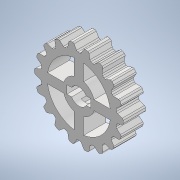
# Autodesk Inventor part: center_gear
Saved by Autodesk Inventor 2022 (Build 260153000, 153)
## iProperties
Created: 2022-06-21
Part Number: center_gear
Material: Generic
Document SubType Name: Modeling
Designer: efred
Density: 1 g/cm^3
Appearance: Default
Author: efred
Autodesk Inventor part; units mm, degrees
ref_plane "YZ Plane" through (0, 0, 0) normal (1, 0, 0) x (0, 1, 0)
ref_plane "XZ Plane" through (0, 0, 0) normal (0, 1, 0) x (-1, 0, 0)
sketch "Sketch1" plane through (0, 0, 0) normal (0, 0, 1) x (1, 0, 0)
  circle A0 centre (0, 0) radius 0.5 projected
  line L0 (-1.1547, -2) -> (-1.7321, -1) projected
  line L1 (-1.7321, -1) -> (-3.5, -1) projected
  line L2 (-3.5, -1) -> (-3.5, 1) projected
  line L3 (-3.5, 1) -> (-1.7321, 1) projected
  line L4 (-1.7321, 1) -> (-1.1547, 2) projected
  line L5 (-1.1547, 2) -> (1.1547, 2) projected
  line L6 (1.1547, 2) -> (1.7321, 1) projected
  line L7 (1.7321, 1) -> (3.5, 1) projected
  line L8 (3.5, 1) -> (3.5, -1) projected
  line L9 (3.5, -1) -> (1.7321, -1) projected
  line L10 (1.7321, -1) -> (1.1547, -2) projected
  line L11 (1.1547, -2) -> (-1.1547, -2) projected
  circle A1 centre (0, 0) radius 5
  line L12 (-3.8, -1.3) -> (-1.9053, -1.3)
  line L13 (-1.9053, -1.3) -> (-1.3279, -2.3)
  line L14 (-1.3279, -2.3) -> (1.3279, -2.3)
  line L15 (1.3279, -2.3) -> (1.9053, -1.3)
  line L16 (1.9053, -1.3) -> (3.8, -1.3)
  line L17 (3.8, -1.3) -> (3.8, 1.3)
  line L18 (3.8, 1.3) -> (1.9053, 1.3)
  line L19 (1.9053, 1.3) -> (1.3279, 2.3)
  line L20 (1.3279, 2.3) -> (-1.3279, 2.3)
  line L21 (-1.3279, 2.3) -> (-1.9053, 1.3)
  line L22 (-1.9053, 1.3) -> (-3.8, 1.3)
  line L23 (-3.8, 1.3) -> (-3.8, -1.3)
  dimension "d0" = 10
  dimension "d1" = 0.3
  constraints: 24 end point, 1 centre point, 1 coincident, 11 other
  measures "d0" diameter of A1
  measures "d1" distance between parallel lines of L1 L12
extrude "Extrusion1" add sketch "Sketch1" along normal blind 2 and the other way blind 5 contours A1
sketch "Sketch2" plane through (0, 0, -5) normal (0, 0, -1) x (-1, 0, 0)
  circle A0 centre (0, 0) radius 5 projected
  line L0 (3.8, 1.3) -> (3.8, -1.3) projected
  line L1 (3.8, -1.3) -> (1.9053, -1.3) projected
  line L2 (1.9053, -1.3) -> (1.3279, -2.3) projected
  line L3 (1.3279, -2.3) -> (-1.3279, -2.3) projected
  line L4 (-1.3279, -2.3) -> (-1.9053, -1.3) projected
  line L5 (-1.9053, -1.3) -> (-3.8, -1.3) projected
  line L6 (-3.8, -1.3) -> (-3.8, 1.3) projected
  line L7 (-3.8, 1.3) -> (-1.9053, 1.3) projected
  line L8 (-1.9053, 1.3) -> (-1.3279, 2.3) projected
  line L9 (-1.3279, 2.3) -> (1.3279, 2.3) projected
  line L10 (1.3279, 2.3) -> (1.9053, 1.3) projected
  line L11 (1.9053, 1.3) -> (3.8, 1.3) projected
  line L12 (3.8, 1.3) -> (3.8, -1.3) projected
  line L13 (3.8, 1.3) -> (3.8, -1.3)
  line L14 (3.8, -1.3) -> (1.9053, -1.3)
  line L15 (1.9053, -1.3) -> (1.3279, -2.3) projected
  line L16 (1.9053, -1.3) -> (1.3279, -2.3)
  line L17 (-1.9053, -1.3) -> (-1.3279, -2.3) projected
  line L18 (-1.3279, -2.3) -> (1.3279, -2.3)
  line L19 (1.9053, 1.3) -> (3.8, 1.3) projected
  line L20 (3.8, 1.3) -> (1.9053, 1.3)
  line L21 (1.3279, 2.3) -> (1.9053, 1.3) projected
  line L22 (1.9053, 1.3) -> (1.3279, 2.3)
  line L23 (1.3279, 2.3) -> (-1.3279, 2.3)
  line L24 (-1.3, 1.9053) -> (-2.3, 1.3279)
  line L25 (-2.3, 1.3279) -> (-2.3, -1.3279)
  line L26 (2.3, -1.3279) -> (2.3, 1.3279)
  line L27 (1.3, 1.9053) -> (2.3, 1.3279)
  line L28 (1.3, 3.8) -> (1.3, 1.9053)
  line L29 (-1.3, 3.8) -> (-1.3, 1.9053)
  line L30 (-1.3, 3.8) -> (1.3, 3.8)
  line L31 (-1.9053, -1.3) -> (-1.3279, -2.3)
  line L32 (-1.3279, -2.3) -> (1.3279, -2.3)
  line L33 (1.3279, 2.3) -> (-1.3279, 2.3)
  line L34 (-1.9053, 1.3) -> (-1.3279, 2.3)
  line L35 (-3.8, 1.3) -> (-1.9053, 1.3)
  line L36 (-3.8, -1.3) -> (-1.9053, -1.3)
  line L37 (-3.8, -1.3) -> (-3.8, 1.3)
  line L38 (1.3, -1.9053) -> (2.3, -1.3279)
  line L39 (2.3, -1.3279) -> (2.3, 1.3279)
  line L40 (-2.3, 1.3279) -> (-2.3, -1.3279)
  line L41 (-1.3, -1.9053) -> (-2.3, -1.3279)
  line L42 (-1.3, -3.8) -> (-1.3, -1.9053)
  line L43 (1.3, -3.8) -> (1.3, -1.9053)
  line L44 (1.3, -3.8) -> (-1.3, -3.8)
  point P0 (1.3, -2.3)
  point P1 (-1.3, -2.3)
  point P2 (-1.3, 2.3)
  point P3 (1.3, 2.3)
  point P4 (-2.3, 1.3)
  point P5 (-1.6837, 1.6837)
  point P6 (-1.6837, -1.6837)
  point P7 (-2.3, -1.3)
  point P8 (1.6837, -1.6837)
  point P9 (2.3, -1.3)
  point P10 (1.6837, 1.6837)
  point P11 (2.3, 1.3)
  dimension "d8" = 360
  constraints: 56 end point, 4 collinear, 1 point on line, 65 other
ref_plane "Work Plane1" through (-8.8, -2.2, 0) normal (0, 0, 1) x (1, 0, 0)
extrude "Extrusion2" cut sketch "Sketch2" against normal up to surface (5 mm away) contours L11 L10 L27 L26 | L26 L38 L2 L1 | L9 L29 L30 L28 | L43 L44 L42 L3 | L8 L7 L25 L24 | L41 L25 L5 L4
sketch "Sketch3" plane through (0, 0, -5) normal (0, 0, -1) x (-1, 0, 0)
  line L0 (-1.6837, 1.6837) -> (-2.3, 1.3279) projected
  circle A0 centre (0, 0) radius 2.6558
  constraints: 1 coincident, 3 other
extrude "Extrusion3" cut sketch "Sketch3" against normal through all
sketch "Sketch4" plane through (0, 0, -5) normal (0, 0, -1) x (-1, 0, 0)
  circle A0 centre (0, 0) radius 5 projected
  circle A1 centre (0, 0) radius 14.5 construction
  circle A2 centre (-20.3143, -27.9603) radius 16.5 construction
  circle A3 centre (0, 0) radius 12.5
  circle A4 centre (0, 0) radius 10.5
  line L0 (-12.4097, -1.5) -> (-4.7697, -1.5)
  line L1 (-4.7697, -1.5) -> (-4.7697, 1.5)
  line L2 (-4.7697, 1.5) -> (-12.4097, 1.5)
  line L3 (-12.4097, 1.5) -> (-12.4097, -1.5)
  line L4 (-5, 0) -> (-10.5, 0) construction
  line L5 (1.5, -12.4097) -> (1.5, -4.7697)
  line L6 (-1.5, -4.7697) -> (-1.5, -12.4097)
  line L7 (12.4097, 1.5) -> (4.7697, 1.5)
  line L8 (4.7697, -1.5) -> (12.4097, -1.5)
  line L9 (-1.5, 12.4097) -> (-1.5, 4.7697)
  line L10 (1.5, 4.7697) -> (1.5, 12.4097)
  line L11 (-14.1647, -0.8644) -> (-12.4097, -1.5)
  line L12 (-14.1647, 0.8644) -> (-12.4097, 1.5)
  arc A5 (-14.4942, 0.4084) -> (-14.4942, -0.4084) centre (0, 0) ccw
  arc A6 (-14.4942, -0.4084) -> (-14.1647, -0.8644) centre (-13.9944, -0.3943) ccw
  arc A7 (-14.1647, 0.8644) -> (-14.4942, 0.4084) centre (-13.9944, 0.3943) ccw
  arc A8 (-12.695, 1.3967) -> (-12.3705, 1.795) centre (-12.8653, 1.8668) ccw
  arc A9 (-12.3705, -1.795) -> (-12.695, -1.3967) centre (-12.8653, -1.8668) ccw
  arc A10 (-12.4071, -3.0295) -> (-12.2383, -2.5442) centre (-12.7279, -2.646) ccw
  line L13 (-13.6061, -4.0323) -> (-12.1743, -2.8348)
  arc A11 (-13.6061, -4.0323) -> (-13.7598, -4.5736) centre (-13.2853, -4.4159) ccw
  arc A12 (-13.7598, -4.5736) -> (-13.4805, -5.3411) centre (0, 0) ccw
  arc A13 (-13.4805, -5.3411) -> (-13.0148, -5.6569) centre (-13.0156, -5.1569) ccw
  arc A14 (-11.0105, -5.9177) -> (-11.4517, -5.6544) centre (-11.4509, -6.1544) ccw
  line L14 (-13.0148, -5.6569) -> (-11.1482, -5.6539)
  arc A15 (-10.6227, -7.0903) -> (-10.6301, -6.5765) centre (-11.0553, -6.8396) ccw
  line L15 (-11.4064, -8.4427) -> (-10.4705, -6.8277)
  arc A16 (-11.4064, -8.4427) -> (-11.3657, -9.0039) centre (-10.9738, -8.6934) ccw
  arc A17 (-11.3657, -9.0039) -> (-10.8407, -9.6295) centre (0, 0) ccw
  arc A18 (-10.8407, -9.6295) -> (-10.2952, -9.7671) centre (-10.4669, -9.2975) ccw
  arc A19 (-8.3225, -9.3266) -> (-8.8272, -9.2301) centre (-8.6554, -9.6997) ccw
  line L16 (-10.2952, -9.7671) -> (-8.5422, -9.1259)
  arc A20 (-7.5571, -10.2959) -> (-7.7397, -9.8156) centre (-8.0493, -10.2083) ccw
  line L17 (-7.8309, -11.8348) -> (-7.5039, -9.9971)
  arc A21 (-7.8309, -11.8348) -> (-7.6008, -12.3482) centre (-7.3387, -11.9224) ccw
  arc A22 (-7.6008, -12.3482) -> (-6.8935, -12.7566) centre (0, 0) ccw
  arc A23 (-6.8935, -12.7566) -> (-6.3338, -12.6992) centre (-6.6558, -12.3167) ccw
  arc A24 (-4.6307, -11.6106) -> (-5.138, -11.6925) centre (-4.816, -12.075) ccw
  line L18 (-6.3338, -12.6992) -> (-4.9058, -11.4971)
  arc A25 (-3.5799, -12.2596) -> (-3.9158, -11.8708) centre (-4.0725, -12.3457) ccw
  line L19 (-3.3109, -13.7994) -> (-3.6321, -11.9607)
  arc A26 (-3.3109, -13.7994) -> (-2.9191, -14.2031) centre (-2.8184, -13.7134) ccw
  arc A27 (-2.9191, -14.2031) -> (-2.1147, -14.345) centre (0, 0) ccw
  arc A28 (-2.1147, -14.345) -> (-1.6084, -14.0996) centre (-2.0418, -13.8503) ccw
  arc A29 (-0.3804, -12.4942) -> (-0.829, -12.7447) centre (-0.3956, -12.994) ccw
  line L20 (-1.6084, -14.0996) -> (-0.6777, -12.4816)
  arc A30 (0.829, -12.7447) -> (0.3804, -12.4942) centre (0.3956, -12.994) ccw
  line L21 (1.6084, -14.0996) -> (0.6777, -12.4816)
  arc A31 (1.6084, -14.0996) -> (2.1147, -14.345) centre (2.0418, -13.8503) ccw
  arc A32 (2.1147, -14.345) -> (2.9191, -14.2031) centre (0, 0) ccw
  arc A33 (2.9191, -14.2031) -> (3.3109, -13.7994) centre (2.8184, -13.7134) ccw
  arc A34 (3.9158, -11.8708) -> (3.5799, -12.2596) centre (4.0725, -12.3457) ccw
  line L22 (3.3109, -13.7994) -> (3.6321, -11.9607)
  arc A35 (5.138, -11.6925) -> (4.6307, -11.6106) centre (4.816, -12.075) ccw
  line L23 (6.3338, -12.6992) -> (4.9058, -11.4971)
  arc A36 (6.3338, -12.6992) -> (6.8935, -12.7566) centre (6.6558, -12.3167) ccw
  arc A37 (6.8935, -12.7566) -> (7.6008, -12.3482) centre (0, 0) ccw
  arc A38 (7.6008, -12.3482) -> (7.8309, -11.8348) centre (7.3387, -11.9224) ccw
  arc A39 (7.7397, -9.8156) -> (7.5571, -10.2959) centre (8.0493, -10.2083) ccw
  line L24 (7.8309, -11.8348) -> (7.5039, -9.9971)
  arc A40 (8.8272, -9.2301) -> (8.3225, -9.3266) centre (8.6554, -9.6997) ccw
  line L25 (10.2952, -9.7671) -> (8.5422, -9.1259)
  arc A41 (10.2952, -9.7671) -> (10.8407, -9.6295) centre (10.4669, -9.2975) ccw
  arc A42 (10.8407, -9.6295) -> (11.3657, -9.0039) centre (0, 0) ccw
  arc A43 (11.3657, -9.0039) -> (11.4064, -8.4427) centre (10.9738, -8.6934) ccw
  arc A44 (10.6301, -6.5765) -> (10.6227, -7.0903) centre (11.0553, -6.8396) ccw
  line L26 (11.4064, -8.4427) -> (10.4705, -6.8277)
  arc A45 (11.4517, -5.6544) -> (11.0105, -5.9177) centre (11.4509, -6.1544) ccw
  line L27 (13.0148, -5.6569) -> (11.1482, -5.6539)
  arc A46 (13.0148, -5.6569) -> (13.4805, -5.3411) centre (13.0156, -5.1569) ccw
  arc A47 (13.4805, -5.3411) -> (13.7598, -4.5736) centre (0, 0) ccw
  arc A48 (13.7598, -4.5736) -> (13.6061, -4.0323) centre (13.2853, -4.4159) ccw
  arc A49 (12.2383, -2.5442) -> (12.4071, -3.0295) centre (12.7279, -2.646) ccw
  line L28 (13.6061, -4.0323) -> (12.1743, -2.8348)
  arc A50 (12.695, -1.3967) -> (12.3705, -1.795) centre (12.8653, -1.8668) ccw
  line L29 (14.1647, -0.8644) -> (12.4097, -1.5)
  arc A51 (14.1647, -0.8644) -> (14.4942, -0.4084) centre (13.9944, -0.3943) ccw
  arc A52 (14.4942, -0.4084) -> (14.4942, 0.4084) centre (0, 0) ccw
  arc A53 (14.4942, 0.4084) -> (14.1647, 0.8644) centre (13.9944, 0.3943) ccw
  arc A54 (12.3705, 1.795) -> (12.695, 1.3967) centre (12.8653, 1.8668) ccw
  line L30 (14.1647, 0.8644) -> (12.4097, 1.5)
  arc A55 (12.4071, 3.0295) -> (12.2383, 2.5442) centre (12.7279, 2.646) ccw
  line L31 (13.6061, 4.0323) -> (12.1743, 2.8348)
  arc A56 (13.6061, 4.0323) -> (13.7598, 4.5736) centre (13.2853, 4.4159) ccw
  arc A57 (13.7598, 4.5736) -> (13.4805, 5.3411) centre (0, 0) ccw
  arc A58 (13.4805, 5.3411) -> (13.0148, 5.6569) centre (13.0156, 5.1569) ccw
  arc A59 (11.0105, 5.9177) -> (11.4517, 5.6544) centre (11.4509, 6.1544) ccw
  line L32 (13.0148, 5.6569) -> (11.1482, 5.6539)
  arc A60 (10.6227, 7.0903) -> (10.6301, 6.5765) centre (11.0553, 6.8396) ccw
  line L33 (11.4064, 8.4427) -> (10.4705, 6.8277)
  arc A61 (11.4064, 8.4427) -> (11.3657, 9.0039) centre (10.9738, 8.6934) ccw
  arc A62 (11.3657, 9.0039) -> (10.8407, 9.6295) centre (0, 0) ccw
  arc A63 (10.8407, 9.6295) -> (10.2952, 9.7671) centre (10.4669, 9.2975) ccw
  arc A64 (8.3225, 9.3266) -> (8.8272, 9.2301) centre (8.6554, 9.6997) ccw
  line L34 (10.2952, 9.7671) -> (8.5422, 9.1259)
  arc A65 (7.5571, 10.2959) -> (7.7397, 9.8156) centre (8.0493, 10.2083) ccw
  line L35 (7.8309, 11.8348) -> (7.5039, 9.9971)
  arc A66 (7.8309, 11.8348) -> (7.6008, 12.3482) centre (7.3387, 11.9224) ccw
  arc A67 (7.6008, 12.3482) -> (6.8935, 12.7566) centre (0, 0) ccw
  arc A68 (6.8935, 12.7566) -> (6.3338, 12.6992) centre (6.6558, 12.3167) ccw
  arc A69 (4.6307, 11.6106) -> (5.138, 11.6925) centre (4.816, 12.075) ccw
  line L36 (6.3338, 12.6992) -> (4.9058, 11.4971)
  arc A70 (3.5799, 12.2596) -> (3.9158, 11.8708) centre (4.0725, 12.3457) ccw
  line L37 (3.3109, 13.7994) -> (3.6321, 11.9607)
  arc A71 (3.3109, 13.7994) -> (2.9191, 14.2031) centre (2.8184, 13.7134) ccw
  arc A72 (2.9191, 14.2031) -> (2.1147, 14.345) centre (0, 0) ccw
  arc A73 (2.1147, 14.345) -> (1.6084, 14.0996) centre (2.0418, 13.8503) ccw
  arc A74 (0.3804, 12.4942) -> (0.829, 12.7447) centre (0.3956, 12.994) ccw
  line L38 (1.6084, 14.0996) -> (0.6777, 12.4816)
  arc A75 (-0.829, 12.7447) -> (-0.3804, 12.4942) centre (-0.3956, 12.994) ccw
  line L39 (-1.6084, 14.0996) -> (-0.6777, 12.4816)
  arc A76 (-1.6084, 14.0996) -> (-2.1147, 14.345) centre (-2.0418, 13.8503) ccw
  arc A77 (-2.1147, 14.345) -> (-2.9191, 14.2031) centre (0, 0) ccw
  arc A78 (-2.9191, 14.2031) -> (-3.3109, 13.7994) centre (-2.8184, 13.7134) ccw
  arc A79 (-3.9158, 11.8708) -> (-3.5799, 12.2596) centre (-4.0725, 12.3457) ccw
  line L40 (-3.3109, 13.7994) -> (-3.6321, 11.9607)
  arc A80 (-5.138, 11.6925) -> (-4.6307, 11.6106) centre (-4.816, 12.075) ccw
  line L41 (-6.3338, 12.6992) -> (-4.9058, 11.4971)
  arc A81 (-6.3338, 12.6992) -> (-6.8935, 12.7566) centre (-6.6558, 12.3167) ccw
  arc A82 (-6.8935, 12.7566) -> (-7.6008, 12.3482) centre (0, 0) ccw
  arc A83 (-7.6008, 12.3482) -> (-7.8309, 11.8348) centre (-7.3387, 11.9224) ccw
  arc A84 (-7.7397, 9.8156) -> (-7.5571, 10.2959) centre (-8.0493, 10.2083) ccw
  line L42 (-7.8309, 11.8348) -> (-7.5039, 9.9971)
  arc A85 (-8.8272, 9.2301) -> (-8.3225, 9.3266) centre (-8.6554, 9.6997) ccw
  line L43 (-10.2952, 9.7671) -> (-8.5422, 9.1259)
  arc A86 (-10.2952, 9.7671) -> (-10.8407, 9.6295) centre (-10.4669, 9.2975) ccw
  arc A87 (-10.8407, 9.6295) -> (-11.3657, 9.0039) centre (0, 0) ccw
  arc A88 (-11.3657, 9.0039) -> (-11.4064, 8.4427) centre (-10.9738, 8.6934) ccw
  arc A89 (-10.6301, 6.5765) -> (-10.6227, 7.0903) centre (-11.0553, 6.8396) ccw
  line L44 (-11.4064, 8.4427) -> (-10.4705, 6.8277)
  arc A90 (-11.4517, 5.6544) -> (-11.0105, 5.9177) centre (-11.4509, 6.1544) ccw
  line L45 (-13.0148, 5.6569) -> (-11.1482, 5.6539)
  arc A91 (-13.0148, 5.6569) -> (-13.4805, 5.3411) centre (-13.0156, 5.1569) ccw
  arc A92 (-13.4805, 5.3411) -> (-13.7598, 4.5736) centre (0, 0) ccw
  arc A93 (-13.7598, 4.5736) -> (-13.6061, 4.0323) centre (-13.2853, 4.4159) ccw
  arc A94 (-12.2383, 2.5442) -> (-12.4071, 3.0295) centre (-12.7279, 2.646) ccw
  line L46 (-13.6061, 4.0323) -> (-12.1743, 2.8348)
  arc A95 (-24.387, -30.8608) -> (-20.267, -32.96) centre (-20.3143, -27.9603) ccw projected
  point P0 (-14.4806, -0.75)
  point P1 (-14.4806, 0.75)
  point P2 (-14.4733, 0.8788)
  point P3 (-12.4097, 1.5)
  point P4 (-12.4097, 1.5)
  point P5 (-12.1743, -2.8348)
  point P6 (-11.1482, -5.6539)
  point P7 (-10.4705, -6.8277)
  point P8 (-8.5422, -9.1259)
  point P9 (-7.5039, -9.9971)
  point P10 (-4.9058, -11.4971)
  point P11 (-3.6321, -11.9607)
  point P12 (-0.6777, -12.4816)
  point P13 (0.6777, -12.4816)
  point P14 (3.6321, -11.9607)
  point P15 (4.9058, -11.4971)
  point P16 (7.5039, -9.9971)
  point P17 (8.5422, -9.1259)
  point P18 (10.4705, -6.8277)
  point P19 (11.1482, -5.6539)
  point P20 (12.1743, -2.8348)
  point P21 (12.4097, 1.5)
  point P22 (12.1743, 2.8348)
  point P23 (11.1482, 5.6539)
  point P24 (10.4705, 6.8277)
  point P25 (8.5422, 9.1259)
  point P26 (7.5039, 9.9971)
  point P27 (3.6321, 11.9607)
  point P28 (0.6777, 12.4816)
  point P29 (-0.6777, 12.4816)
  point P30 (-3.6321, 11.9607)
  point P31 (-4.9058, 11.4971)
  point P32 (-7.5039, 9.9971)
  point P33 (-8.5422, 9.1259)
  point P34 (-10.4705, 6.8277)
  point P35 (-11.1482, 5.6539)
  point P36 (-12.1743, 2.8348)
  point P37 (-10.3923, 1.5)
  point P38 (-1.5, 10.3923)
  point P39 (-1.5, 4.7697)
  point P40 (1.5, 10.3923)
  point P41 (10.3923, 1.5)
  point P42 (4.7697, 1.5)
  point P43 (10.3923, -1.5)
  point P44 (1.5, -10.3923)
  point P45 (1.5, -4.7697)
  point P46 (-1.5, -10.3923)
  point P47 (-10.3923, -1.5)
  point P48 (-12.2383, -2.5442)
  point P49 (-11.4517, -5.6544)
  point P50 (-10.6301, -6.5765)
  point P51 (-8.3225, -9.3266)
  point P52 (-7.7397, -9.8156)
  point P53 (-5.138, -11.6925)
  point P54 (-4.6307, -11.6106)
  point P55 (-3.9158, -11.8708)
  point P56 (-0.829, -12.7447)
  point P57 (-0.3804, -12.4942)
  point P58 (0.3804, -12.4942)
  point P59 (3.9158, -11.8708)
  point P60 (4.6307, -11.6106)
  point P61 (8.3225, -9.3266)
  point P62 (7.5571, -10.2959)
  point P63 (7.7397, -9.8156)
  point P64 (10.6227, -7.0903)
  point P65 (10.6301, -6.5765)
  point P66 (11.0105, -5.9177)
  point P67 (12.3705, -1.795)
  point P68 (12.4071, -3.0295)
  point P69 (12.2383, -2.5442)
  point P70 (12.3705, 1.795)
  point P71 (11.4517, 5.6544)
  point P72 (11.0105, 5.9177)
  point P73 (8.8272, 9.2301)
  point P74 (8.3225, 9.3266)
  point P75 (7.7397, 9.8156)
  point P76 (5.138, 11.6925)
  point P77 (4.6307, 11.6106)
  point P78 (3.9158, 11.8708)
  point P79 (0.829, 12.7447)
  point P80 (0.3804, 12.4942)
  point P81 (-0.3804, 12.4942)
  point P82 (-3.5799, 12.2596)
  point P83 (-3.9158, 11.8708)
  point P84 (-4.6307, 11.6106)
  point P85 (-7.5571, 10.2959)
  point P86 (-7.7397, 9.8156)
  point P87 (-8.3225, 9.3266)
  point P88 (-10.6227, 7.0903)
  point P89 (-10.6301, 6.5765)
  point P90 (-12.4071, 3.0295)
  point P91 (-12.695, -1.3967)
  dimension "d17" = 2
  dimension "d14" = 33
  dimension "d15" = 29
  dimension "d16" = 2
  dimension "d18" = 3
  dimension "d21" = 360
  dimension "d23" = 1.5
  dimension "d24" = 3
  dimension "d25" = 0.5
  dimension "d26" = 0.5
  dimension "d29" = 360
  constraints: 187 point on circle, 94 end point, 92 centre point, 20 point on line, 5 symmetric about line, 5 tangent, 2 coincident, 2 equal radius, 2 horizontal, 2 parallel, 1 horizontal alignment, 1 perpendicular, 431 other
  measures "d14" diameter of A2
  measures "d15" diameter of A1
  measures "d18" distance between parallel lines of L0 L2
  measures "d23" distance of point (-14.481, 0.75) A1.start
  measures "d24" distance of L11.end L12.end
  measures "d25" radius of A6
  measures "d26" radius of A8
extrude "Extrusion4" add sketch "Sketch4" against normal up to surface (7 mm away) contours A0 L7 A4 L8 | A0 L9 A4 L10 | L7 A3 L8 A4 | A4 L10 A3 L7 | L5 A4 L6 A0 | L8 A3 L5 A4 | A4 L9 A3 L10 | L30 A53 A52 A51 L29 A3 | A3 A54 L30 | L5 A3 L6 A4 | L29 A50 A3 | A0 L0 A4 L2 | A4 L2 A3 L9 | A3 L38 A73 A72 A71 L37 | L6 A3 L0 A4 | A3 L22 A33 A32 A31 L21 | A4 L0 L3 L2 | A3 L40 A78 A77 A76 L39 | L37 A70 A3 | A3 A74 L38 | A3 L31 A55 | A3 L20 A28 A27 A26 L19 | L21 A30 A3 | A3 A34 L22 | A49 L28 A3 | L12 A8 A3 | L3 A3 | A3 L11 A6 A5 A7 L12 | L39 A75 A3 | A3 A79 L40 | A3 L32 A58 A57 A56 L31 | A3 A9 L11 | L19 A25 A3 | A3 A29 L20 | L28 A48 A47 A46 L27 A3 | A69 L36 A3 | A3 A59 L32 | A3 L23 A35 | L27 A45 A3 | A94 L46 A3 | A3 L41 A80 | L36 A68 A67 A66 L35 A3 | A3 L13 A10 | A24 L18 A3 | A3 L24 A38 A37 A36 L23 | L46 A93 A92 A91 L45 A3 | A3 L42 A83 A82 A81 L41 | L35 A65 A3 | A3 L33 A60 | A3 L14 A13 A12 A11 L13 | L18 A23 A22 A21 L17 A3 | A3 A39 L24 | A44 L26 A3 | L45 A90 A3 | A3 A84 L42 | A3 L34 A63 A62 A61 L33 | A3 A14 L14 | L17 A20 A3 | L26 A43 A42 A41 L25 A3 | A64 L34 A3 | A3 L25 A40 | A89 L44 A3 | A3 L43 A85 | A3 L15 A15 | A19 L16 A3 | L44 A88 A87 A86 L43 A3 | A3 L16 A18 A17 A16 L15
body "Solid1"
